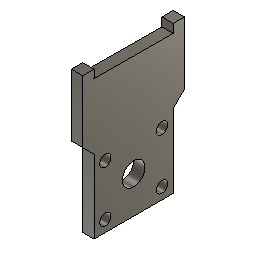
EIXO Z v1 (Autodesk Fusion 360 design; units mm, degrees)
Autodesk Fusion 360 part; units mm, degrees
sketch "Sketch1" plane through (0, 0, 0) normal (1, 0, 0) x (0, 1, 0)
  line L0 (0, 0) -> (-90, 0)
  line L1 (-90, 130) -> (0, 130)
  line L2 (-80, 55) -> (-10, 55) construction
  line L3 (-10, 65) -> (-0.2651, 74.7349)
  line L4 (-80, 65) -> (-90.2415, 75.2415)
  line L5 (-80, 65) -> (-65.5164, 65) construction
  line L6 (-90, 75) -> (-90, 130)
  line L7 (-80, 65) -> (-10, 65)
  line L8 (-10, 65) -> (-5, 65)
  line L9 (-80, 65) -> (-80, 0)
  line L10 (-70, 65) -> (-70, 0) construction
  line L11 (-20, 65) -> (-20, 0) construction
  line L12 (-10, 65) -> (-10, 0)
  line L13 (0, 130) -> (-0.2651, 74.7349)
  line L14 (-80, 10) -> (-10, 10) construction
  line L15 (-70, 32.5) -> (-20, 32.5) construction
  line L16 (-45, 65) -> (-45, 0) construction
  circle A0 centre (-45, 32.5) radius 10
  circle A1 centre (-70, 55) radius 5
  circle A2 centre (-70, 10) radius 5
  circle A3 centre (-20, 55) radius 5
  circle A4 centre (-20, 10) radius 5
  line L17 (-90, 130) -> (-80, 130) construction
  line L18 (0, 130) -> (12.7629, 130) construction
  line L19 (-10, 130) -> (-10, 122.4135)
  line L20 (-80, 130) -> (-80.0348, 122.7494)
  line L21 (-80.0348, 122.7494) -> (-10, 122.4135)
  dimension "d1" = 90
  dimension "d2" = 130
  dimension "d10" = 65
  dimension "d16" = 45
  dimension "d17" = 135
  dimension "d20" = 10
  dimension "d22" = 10
  dimension "d26" = 10
  dimension "d27" = 35
  dimension "d28" = 20
  dimension "d29" = 10
  dimension "d30" = 10
  dimension "d31" = 10
  dimension "d32" = 10
  dimension "d37" = 10
  dimension "d39" = 10
  constraint horizontal L0
  constraint horizontal L1
  constraint coincident L0.start origin
  constraint coincident L0 L12.end
  constraint coincident L0 L9.end
  constraint horizontal L8
  constraint horizontal L5
  constraint coincident L5 L10.start
  constraint coincident L7 L10.start
  constraint coincident L0 L10.end
  constraint perpendicular L0 L10
  constraint coincident L7 L11.start
  constraint coincident L0 L11.end
  constraint perpendicular L0 L11
  constraint coincident L4 L6.start
  constraint coincident L9 L14.start
  constraint coincident L12 L14.end
  constraint perpendicular L12 L14
  constraint midpoint L10 L15.start
  constraint midpoint L11 L15.end
  constraint coincident L7 L16.start
  constraint coincident L0 L16.end
  constraint perpendicular L0 L16
  constraint midpoint L16 A0.centre
  constraint coincident L10 A1.centre
  constraint coincident L2 A1.centre
  constraint coincident L14 A2.centre
  constraint coincident L10 A2.centre
  constraint coincident L2 A3.centre
  constraint coincident L11 A3.centre
  constraint coincident L14 A4.centre
  constraint coincident L11 A4.centre
  constraint horizontal L17
  constraint horizontal L18
  constraint coincident L1 L19.start
  constraint perpendicular L1 L19
  measures "d1" distance of L0.start L0.end
  measures "d2" distance of L0.start L1.end
  measures "d10" distance of L0 L7
  measures "d16" angle of L3 L8
  measures "d17" angle of L4 L5
  measures "d20" distance of L9 L10
  measures "d22" distance of L2.end L3.start
  measures "d26" distance of L0 L14
  measures "d27" distance of L9 L16
  measures "d28" diameter of A0
  measures "d29" diameter of A1
  measures "d30" diameter of A2
  measures "d31" diameter of A3
  measures "d32" diameter of A4
  measures "d37" distance of L1.start L17.end
  measures "d39" distance of L1.end L19
extrude "Extrude1" add sketch "Sketch1" against normal blind 10 contours L0 L7 L9 L12 | L1 L3 L4 L6 L7 L13 L19 L20 L21 | A0 | A1 | A2 | A3 | A4
extrude "Extrude2" cut sketch "Sketch1" against normal blind 10 contours A0 | A1 | A2 | A3 | A4
